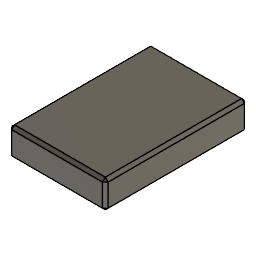
Main (Autodesk Fusion 360 archive; units mm, degrees)
design "Batery"
Autodesk Fusion 360 part; units mm, degrees
sketch "Sketch1" plane through (0, 0, 0) normal (0, 0, 1) x (1, 0, 0)
  line L0 (0, 0) -> (34, 0)
  line L1 (34, 0) -> (34, 50)
  line L2 (34, 50) -> (0, 50)
  line L3 (0, 50) -> (0, 0)
  dimension "d1" = 34
  dimension "d2" = 50
  constraint horizontal L0
  constraint vertical L1
  constraint horizontal L2
  constraint vertical L3
  constraint coincident L0.start L3.end
  measures "d1" distance of L0.start L0.end
  measures "d2" distance of L0.start L2.end
extrude "Extrude1" add sketch "Sketch1" along normal blind 10
chamfer "Chamfer1" distance 1 distance2 1 6 faces at (11.3333, 33.3333, 10) (11.3333, 33.3333, 0) (34, 16.6667, 3.3333) (11.3333, 0, 3.3333) (0, 33.3333, 3.3333) (22.6667, 50, 3.3333)

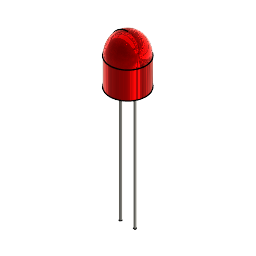
design "LED"
Autodesk Fusion 360 part; units mm, degrees
sketch "Sketch1" plane through (0, 0, 0) normal (0, 0, 1) x (1, 0, 0)
  circle A0 centre (0, 0) radius 1.5
  constraint coincident A0.centre origin
extrude "Extrude1" add sketch "Sketch1" along normal blind 4
fillet "Fillet1" offset 1.49 second offset 1.75 1 edges at (-1.3985, -0.5424, 4) measured on face at (-0.4452, -0.0508, 4)
sketch "Sketch2" plane through (0, 0, 0) normal (0, 0, -1) x (1, 0, 0)
  circle A0 centre (0, 0) radius 1.5
  circle A1 centre (0.6, 0) radius 0.1
  circle A2 centre (-0.6, 0) radius 0.1
extrude "Extrude2" add sketch "Sketch2" along normal blind 10 contours A1 | A2
